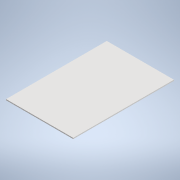
# Autodesk Inventor part: ramp
Saved by Autodesk Inventor 2021 (Build 250183000, 183)
## iProperties
Created: 2020-09-12
Part Number: ramp
Material: Generic
Document SubType Name: Modeling
Designer: deli
Density: 1 g/cm^3
Appearance: Default
Author: deli
Autodesk Inventor part; units mm, degrees
ref_plane "YZ Plane" through (0, 0, 0) normal (1, 0, 0) x (0, 1, 0)
ref_plane "XZ Plane" through (0, 0, 0) normal (0, 1, 0) x (-1, 0, 0)
ref_plane "XY Plane" through (0, 0, 0) normal (0, 0, 1) x (1, 0, 0)
sketch "Sketch1" plane through (0, 0, 0) normal (0, 1, 0) x (-1, 0, 0)
  line L0 (56.1087, 112.1187) -> (-147.0913, 112.1187)
  line L1 (-147.0913, 112.1187) -> (-147.0913, -192.6813)
  line L2 (-147.0913, -192.6813) -> (56.1087, -192.6813)
  line L3 (56.1087, -192.6813) -> (56.1087, 112.1187)
  point P0 (0, 0)
  dimension "d2" = 304.8
  dimension "d3" = 203.2
  constraints: 8 end point, 2 parallel, 1 horizontal, 1 perpendicular
  measures "d2" distance of L2.end L0.start
  measures "d3" distance of L0.start L0.end
extrude "Extrusion1" add sketch "Sketch1" along normal blind 3.175
sketch "Sketch2" plane through (0, 3.175, 0) normal (0, 1, 0) x (1, 0, 0)
  circle A0 centre (121.6913, 116.4813) radius 11.43
  line L0 (147.0913, 192.6813) -> (-56.1087, 192.6813) projected
  line L1 (-56.1087, 192.6813) -> (-56.1087, -112.1187) projected
  circle A1 centre (131.5908, 106.5818) radius 1.25 projected
  circle A2 centre (131.5908, 126.3808) radius 1.25 projected
  circle A3 centre (111.7918, 106.5818) radius 1.25 projected
  circle A4 centre (111.7918, 126.3808) radius 1.25 projected
  point P0 (0, 0)
  dimension "d4" = 22.86
  dimension "d5" = 76.2
  dimension "d6" = 177.8
  constraints: 1 centre point
  measures "d4" diameter of A0
  measures "d5" distance from line of L0 A0.centre
  measures "d6" distance from line of A0.centre L1
extrude "Extrusion2" cut sketch "Sketch2" against normal blind 25.4
body "Solid1"
